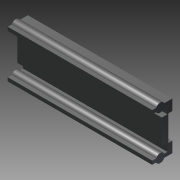
# Autodesk Inventor part: BSPG-SL1560Retainer
Saved by Autodesk Inventor 2016 (Build 200138000, 138)
## iProperties
Category: PARTsolutions
Company: IKO
Created: 2015-05-07
Part Number: BSPG-SL1560Retainer
Catalog Web Link: www.cadenas.de
Description: BSPG - Retainer-
Vendor: IKO
Document SubType Name: Modeling
Designer: PARTuser1
Manufacturer: IKO
Mass: 0.97329 g
Surface Area: 17.851 cm^2
Volume: 0.97329 cm^3
Density: 1 g/cm^3
Material: Generic
Appearance: PSOLRGB-192-192-192
PSOL_IDENT_0: {$CADENAS_DATA\23d-libs\iko\linear_way_series\precise_ball_slide\bspg_2.prj},189 {VTYP=3D},{NB=BSPG-
PSOL_IDENT_1: SL1560Retainer},{LINA=BSPG-SL1560Retainer},{NN=BSPG - Retainer},{DATE=18.01.2008 10:02:28},{GEOMDATE=
PSOL_IDENT_2: 05.10.2007 11:12:00},{VERSION=},{LINEID=60},{LINESUBID=-1},{WBVAR=}  {NB=BSPG-SL1560Retainer},{LINA=
PSOL_IDENT_3: BSPG-SL1560Retainer},{KT=DUMMY},{IDNR=},{TP=BSPG-SL},{SZ=15},{L=60.000},{L2=36.000},{W1=11.800},{W2=
PSOL_IDENT_4: 10.000},{W3=6.200},{W4=1.900},{W5=6.000},{H1=5.000},{H2=3.000},{H3=1.000},{H4=2.600},{T1=0.900},{T2=
PSOL_IDENT_5: 1.200},{T3=0.000},{R1=1.000},{R2=0.200},{R3=0.200},{R4=0.200},{A=90.000},{DA=2.200}
SUPPLIER: IKO
ARTICLENO: BSPG-SL1560Retainer
BOMINFO: BSPG-SL1560Retainer
CREATOR: CADENAS GmbH
Title: BSPG-SL1560Retainer
Author: Cadenas PARTsolutions
Autodesk Inventor part; units mm, degrees
ref_plane "YZ Plane" through (0, 0, 0) normal (1, 0, 0) x (0, 1, 0)
ref_plane "XZ Plane" through (0, 0, 0) normal (0, 1, 0) x (-1, 0, 0)
ref_plane "XY Plane" through (0, 0, 0) normal (0, 0, 1) x (1, 0, 0)
sketch "Sketch_1" plane through (0, 0, 0) normal (1, 0, 0) x (0, 1, 0)
  arc A0 (1.0037, 5.9) -> (-1.0037, 5.9) centre (0, 5.45) ccw
  line L0 (-1.0037, 5.9) -> (-2, 5.9)
  line L1 (-2, 5.9) -> (-2, 5)
  line L2 (-2, 5) -> (-1.0037, 5)
  arc A1 (-1.0037, 5) -> (1.0037, 5) centre (0, 5.45) ccw
  line L3 (1.0037, 5) -> (1.8, 5)
  line L4 (1.8, 5) -> (1.8, 3.1)
  line L5 (1.8, 3.1) -> (0.4, 3.1)
  line L6 (0.4, 3.1) -> (0.4, -3.1)
  line L7 (0.4, -3.1) -> (1.8, -3.1)
  line L8 (1.8, -3.1) -> (1.8, -5)
  line L9 (1.8, -5) -> (1.0037, -5)
  arc A2 (1.0037, -5) -> (-1.0037, -5) centre (0, -5.45) ccw
  line L10 (-1.0037, -5) -> (-2, -5)
  line L11 (-2, -5) -> (-2, -5.9)
  line L12 (-2, -5.9) -> (-1.0037, -5.9)
  arc A3 (-1.0037, -5.9) -> (1.0037, -5.9) centre (0, -5.45) ccw
  line L13 (1.0037, -5.9) -> (3, -5.9)
  line L14 (3, -5.9) -> (3, -3.2)
  line L15 (3, -3.2) -> (2, -3.2)
  line L16 (2, -3.2) -> (2, 3.2)
  line L17 (2, 3.2) -> (3, 3.2)
  line L18 (3, 3.2) -> (3, 5.9)
  line L19 (3, 5.9) -> (1.0037, 5.9)
  constraints: 40 end point, 8 point on circle, 4 centre point
extrude "Extrusion1" add sketch "Sketch_1" along normal blind 36
ref_plane "bspg_rt_XY" through (18, 0, 0) normal (1, 0, 0) x (0, 0, -1)
ref_plane "bspg_rt_YZ" through (18, 0, 0) normal (0, 0, -1) x (0, 1, 0)
ref_plane "bspg_rt_ZX" through (18, 0, 0) normal (0, 1, 0) x (1, 0, 0)
body "Solid1"
